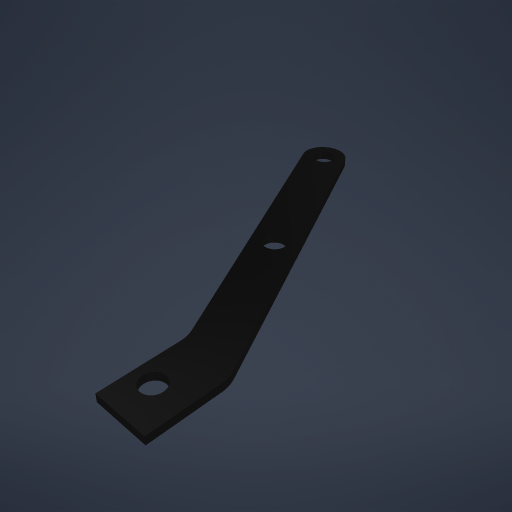
# Autodesk Inventor part: Front Guard
Saved by Autodesk Inventor 2023 (Build 270158000, 158)
## iProperties
Created: 2022-10-29
Part Number: Front Guard
Material: Generic
Document SubType Name: Modeling
Designer: alex
Density: 1 g/cm^3
Appearance: Default
Author: alex
Autodesk Inventor part; units mm, degrees
ref_plane "YZ Plane" through (0, 0, 0) normal (1, 0, 0) x (0, 1, 0)
ref_plane "XZ Plane" through (0, 0, 0) normal (0, 1, 0) x (-1, 0, 0)
ref_plane "XY Plane" through (0, 0, 0) normal (0, 0, 1) x (1, 0, 0)
sketch "Sketch2" plane through (0, 0, 0) normal (0, 1, 0) x (-1, 0, 0)
  arc A0 (-315.9842, -7.0824) -> (-308.3642, -3.3824) centre (-312.1742, -5.2324) ccw
  line L0 (-312.1742, -5.2324) -> (-308.3642, -3.3824) construction
  line L1 (-312.1742, -5.2324) -> (-315.9842, -7.0824) construction
  line L2 (-343.9242, 64.6176) -> (-343.9242, 51.9176)
  line L3 (-343.9242, 64.6176) -> (-343.9242, 53.0352)
  line L4 (-343.9242, 64.6176) -> (-333.7642, 64.6176)
  arc A1 (-343.9242, 51.9176) -> (-343.2864, 49.1439) centre (-337.5742, 51.9176) ccw
  line L5 (-315.9842, -7.0824) -> (-343.2864, 49.1439)
  line L6 (-333.7642, 64.6176) -> (-333.7642, 50.3868)
  arc A2 (-333.7642, 50.3868) -> (-333.1264, 47.6131) centre (-327.4142, 50.3868) ccw
  line L7 (-333.1264, 47.6131) -> (-308.3642, -3.3824)
  circle A3 centre (-337.5742, 58.2676) radius 2.1463
  circle A4 centre (-312.1742, -5.2324) radius 2.1463
  circle A5 centre (-326.0427, 23.3285) radius 2.1463
  point P0 (0, 0)
  dimension "d0" = 180
  dimension "d1" = 3.81
  dimension "d2" = 10.16
  dimension "d3" = 12.7
  dimension "d4" = 6.35
  dimension "d5" = 31.75
  dimension "d6" = 69.85
  dimension "d7" = 6.35
  dimension "d8" = 4.2926
  dimension "d9" = 4.2926
  dimension "d10" = 6.35
  dimension "d11" = 6.35
  dimension "d12" = 4.2926
  dimension "d13" = 31.75
  dimension "d14" = 4.2354
  constraints: 16 end point, 7 point on circle, 6 centre point, 6 tangent, 2 perpendicular, 2 vertical, 1 coincident, 1 collinear
  measures "d0" angle of L0 L1
  measures "d1" horizontal distance of L0.start L1.end
  measures "d2" distance of L2.start L4.end
  measures "d3" distance of L2.start L2.end
  measures "d4" distance from line of A1.centre L2
  measures "d5" distance from line of L2 L0.start
  measures "d6" distance from line of L0.start L4
  measures "d7" distance from line of L6 A2.centre
  measures "d8" diameter of A3
  measures "d9" diameter of A4
  measures "d10" distance from line of A3.centre L4
  measures "d11" distance from line of A3.centre L2
  measures "d12" diameter of A5
  measures "d13" distance of A4.centre A5.centre
  measures "d14" distance from line of L5 A5.centre
extrude "Extrusion1" add sketch "Sketch2" along normal blind 1.5875
body "Solid1"
